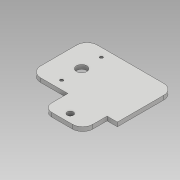
# Autodesk Inventor part: Верт держатели-2 правый
Saved by Autodesk Inventor 2018 (Build 220112000, 112)
## iProperties
Created: 2020-03-15
Part Number: Верт держатели-2 правый
Material: Типовые
Document SubType Name: Modeling
Designer: Leancher
Density: 1 g/cm^3
Appearance: По умолчанию
Author: Leancher
Autodesk Inventor part; units mm, degrees
ref_plane "YZ Plane" through (0, 0, 0) normal (1, 0, 0) x (0, 1, 0)
ref_plane "XZ Plane" through (0, 0, 0) normal (0, 1, 0) x (-1, 0, 0)
ref_plane "XY Plane" through (0, 0, 0) normal (0, 0, 1) x (1, 0, 0)
sketch "Эскиз1" plane through (0, 0, 0) normal (0, 0, 1) x (1, 0, 0)
  arc A0 (-17.4305, 17.6734) -> (-22.4305, 12.6734) centre (-17.4305, 12.6734) ccw
  line L0 (-22.4305, 12.6734) -> (-22.4305, -4.8714)
  arc A1 (-22.4305, -4.8714) -> (-17.4305, -9.8714) centre (-17.4305, -4.8714) ccw
  line L1 (-17.4305, -9.8714) -> (-4.1609, -9.8714)
  line L2 (-4.1609, -9.8714) -> (-4.1609, -17.7214)
  arc A2 (-4.1609, -17.7214) -> (-0.1609, -21.7214) centre (-0.1609, -17.7214) ccw
  line L3 (-0.1609, -21.7214) -> (9.8391, -21.7214)
  arc A3 (9.8391, -21.7214) -> (14.8391, -16.7214) centre (9.8391, -16.7214) ccw
  line L4 (14.8391, -16.7214) -> (14.8391, -9.8714)
  line L5 (19.8391, -9.8714) -> (19.8391, 12.6734)
  arc A4 (19.8391, 12.6734) -> (14.8391, 17.6734) centre (14.8391, 12.6734) ccw
  line L6 (14.8391, 17.6734) -> (-17.4305, 17.6734)
  circle A5 centre (-11.2957, 3.901) radius 2.5
  circle A6 centre (4.8391, -17.7214) radius 1.5
  line L7 (14.8391, -9.8714) -> (19.8391, -9.8714)
  circle A7 centre (-11.2957, 13.465) radius 0.75
  circle A8 centre (-11.2957, -5.8075) radius 0.75
  point P0 (0, 0)
  dimension "d0" = 5
  constraints: 16 end point, 10 point on circle, 9 centre point
  measures "d0" diameter of A5
extrude "Выдавливание1" add sketch "Эскиз1" along normal blind 2
chamfer "Фаска3" distance 2 angle 45 1 edges at (-12.0457, -5.8075, 0)
chamfer "Фаска4" distance 2 angle 45 1 edges at (-12.0457, 13.465, 0)
